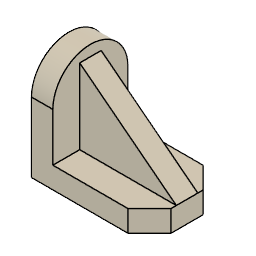
d2-1 (Autodesk Fusion 360 design; units mm, degrees)
part number: 2026-08-20-17-48-57-434
Autodesk Fusion 360 part; units mm, degrees
sketch "Sketch1" plane through (0, 0, 0) normal (0, 1, 0) x (1, 0, 0)
  line L0 (33, 21) -> (-33, 21)
  line L1 (-33, 21) -> (-33, -21)
  line L2 (-33, -21) -> (33, -21)
  line L3 (33, -21) -> (33, 21)
  line L4 (33, 21) -> (-33, -21) construction
  line L5 (-33, 21) -> (33, -21) construction
  dimension "d1" = 66
  dimension "d2" = 42
  constraint horizontal L0
  constraint perpendicular L0 L1
  constraint parallel L0 L2
  constraint parallel L1 L3
  constraint coincident L4 origin
  constraint coincident L5 origin
  measures "d1" distance of L1.end L2.end
  measures "d2" distance of L0.end L1.end
extrude "Extrude1" add sketch "Sketch1" along normal blind 12
chamfer "Chamfer1" distance 12 angle 45 2 edges at (33, 6, 21) (33, 6, -21)
sketch "Sketch2" plane through (-33, 0, 0) normal (-1, 0, 0) x (0, 0, 1)
  line L0 (-21, 0) -> (21, 0)
  line L1 (21, 0) -> (21, 12)
  line L2 (21, 12) -> (-21, 12)
  line L3 (-21, 12) -> (-21, 0)
  line L4 (21, 12) -> (21, 39)
  line L5 (-21, 39) -> (-21, 12)
  line L6 (-21, 12) -> (21, 12)
  arc A0 (21, 39) -> (-21, 39) centre (0, 39) ccw
  dimension "d8" = 42
  dimension "d9" = 27
  constraint coincident L1.end L2.start
  constraint perpendicular L2 L4
  constraint coincident L2.end L3.start
  measures "d8" diameter of A0
  measures "d9" distance of L6 A0.centre
extrude "Extrude2" add sketch "Sketch2" against normal blind 12 contours L2 L4 L5 L6 A0
sketch "Sketch3" plane through (-21, 0, 0) normal (1, 0, 0) x (0, 0, -1)
  arc A0 (21, 39) -> (-21, 39) centre (0, 39) ccw
  line L0 (-21, 39) -> (-21, 12)
  line L1 (-21, 12) -> (21, 12)
  line L2 (21, 12) -> (21, 39)
  line L3 (-6, 12) -> (-6, 54)
  line L4 (-6, 54) -> (6, 54)
  line L5 (6, 54) -> (6, 12)
  dimension "d12" = 42
  dimension "d13" = 15
  dimension "d14" = 12
  dimension "d15" = 42
  constraint coincident L1 L3.start
  constraint perpendicular L1 L3
  constraint perpendicular L3 L4
  constraint perpendicular L4 L5
  measures "d12" distance of L3.start L3.end
  measures "d13" distance of L0.end L3.start
  measures "d14" distance of L3.end L4.end
  measures "d15" distance of L4.end L5.end
extrude "Extrude3" add sketch "Sketch3" along normal blind 54 contours L1 L3 L4 L5
sketch "Sketch4" plane through (0, 0, 6) normal (0, 0, 1) x (1, 0, 0)
  line L0 (-21, 54) -> (-21, 12)
  line L1 (-21, 12) -> (33, 12)
  line L2 (33, 12) -> (33, 54)
  line L3 (33, 54) -> (-21, 54)
  line L4 (33, 12) -> (-21, 54)
  line L5 (33, 12) -> (33, 54)
  line L6 (-21, 54) -> (33, 54)
  constraint coincident L1.end L2.start
  constraint coincident L0.start L3.end
  constraint coincident L2.end L3.start
extrude "Extrude4" cut sketch "Sketch4" against normal blind 12 contours L2 L3 L4 L5 L6
